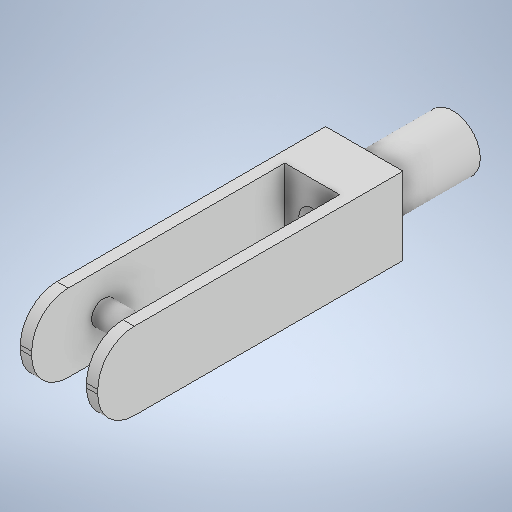
# Autodesk Inventor part: G
Saved by Autodesk Inventor 2025.3 (Build 293356000, 356)
## iProperties
Created: 2025-07-14
Part Number: G
Material: Generic
Document SubType Name: Modeling
Designer: steve
Density: 1 g/cm^3
Appearance: Default
Author: steve
Autodesk Inventor part; units mm, degrees
ref_plane "YZ Plane" through (0, 0, 0) normal (1, 0, 0) x (0, 1, 0)
ref_plane "XZ Plane" through (0, 0, 0) normal (0, 1, 0) x (-1, 0, 0)
ref_plane "XY Plane" through (0, 0, 0) normal (0, 0, 1) x (1, 0, 0)
sketch "Sketch1" plane through (0, 0, 0) normal (0, 0, 1) x (1, 0, 0)
  circle A0 centre (0, 0) radius 0.95
  circle A1 centre (0, 0) radius 1.95
  dimension "d0" = 1.9
  dimension "d1" = 3.9
  constraints: 2 centre point, 2 coincident
  measures "d0" diameter of A0
  measures "d1" diameter of A1
extrude "Extrusion1" add sketch "Sketch1" along normal blind 6.3
sketch "Sketch2" plane through (0, 0, 6.3) normal (0, 0, 1) x (1, 0, 0)
  line L0 (-2.75, -2.75) -> (2.75, -2.75)
  line L1 (2.75, -2.75) -> (2.75, 2.75)
  line L2 (2.75, 2.75) -> (-2.75, 2.75)
  line L3 (-2.75, 2.75) -> (-2.75, -2.75)
  line L4 (-2.75, -2.75) -> (2.75, 2.75) construction
  line L5 (2.75, -2.75) -> (-2.75, 2.75) construction
  point P0 (0, 0)
  dimension "d4" = 5.5
  dimension "d5" = 5.5
  constraints: 12 end point, 2 midpoint, 2 parallel, 1 horizontal, 1 perpendicular
  measures "d4" distance of L2.end L1.end
  measures "d5" distance of L1.end L0.end
extrude "Extrusion2" add sketch "Sketch2" along normal blind 3.7
extrude "Extrusion3" cut sketch "Sketch1" along normal through all contours A0
sketch "Sketch3" plane through (-2.75, 2.75, 6.3) normal (0, 1, 0) x (1, 0, 0)
  line L0 (0.8, 6.3) -> (0.8, 0) projected
  line L1 (0, 0) -> (0, -3.7) projected
  line L2 (0, -3.7) -> (5.5, -3.7) projected
  line L3 (0, -3.7) -> (0.8, -3.7)
  line L4 (6.7827, -4.1433) -> (6.7693, -4.1433)
  line L5 (0.8, -3.7) -> (0.8, -21.7)
  line L6 (0.8, -21.7) -> (0, -21.7)
  line L7 (0, -21.7) -> (0, -3.7)
  line L8 (2.75, -3.7) -> (2.75, -2.5481)
  line L9 (4.7, -3.7) -> (4.7, -21.7)
  line L10 (4.7, -21.7) -> (5.5, -21.7)
  line L11 (5.5, -21.7) -> (5.5, -3.7)
  point P0 (2.75, 6.3)
  dimension "d10" = 18
  constraints: 18 end point, 3 symmetric about line, 2 vertical, 1 collinear, 1 horizontal, 1 midpoint, 1 perpendicular, 1 point on line
  measures "d10" distance of L3.end L5.end
extrude "Extrusion4" add sketch "Sketch3" against normal up to surface (5.5 mm away)
sketch "Sketch4" plane through (-2.75, -2.75, 6.3) normal (-1, 0, 0) x (0, 0, 1)
  line L0 (21.7, 5.5) -> (21.7, 0) projected
  line L1 (21.7, 2.75) -> (19.1, 2.75)
  circle A0 centre (16.5832, 2.75) radius 0.86
  point P0 (-6.3, 2.75)
  dimension "d13" = 2.6
  dimension "d14" = 1.72
  constraints: 2 end point, 1 centre point, 1 horizontal, 1 midpoint
  measures "d13" distance of L1.start L1.end
  measures "d14" diameter of A0
extrude "Extrusion5" add sketch "Sketch4" against normal up to surface (5.5 mm away)
fillet "Fillet1" radius 2.6 2 edges at (-2.35, -2.75, 28) (-2.35, 2.75, 28)
fillet "Fillet2" radius 2.6 2 edges at (2.35, 2.75, 28) (2.35, -2.75, 28)
body "Solid1"
